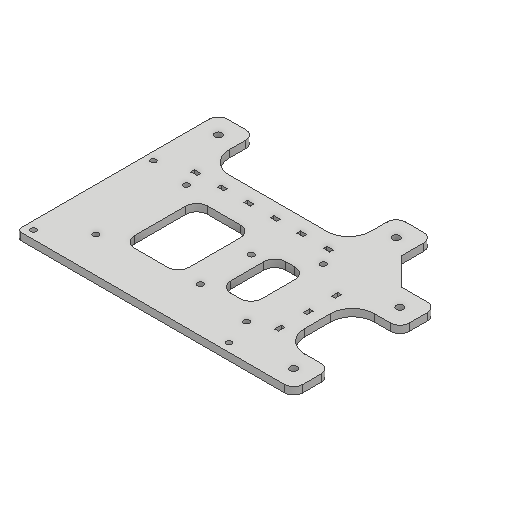
# Autodesk Inventor part: 3DP_PLA_Controller_Case_Bottom
Saved by Autodesk Inventor 2026.1 (Build 301233000, 233)
## iProperties
Created: 2017-05-26
Part Number: 3DP_PLA_Controller_Case_Bottom
Material: Ogólny
Document SubType Name: Modeling
Designer: Andrzej
Density: 1 g/cm^3
Appearance: Domyślna
Mass: 43.8091 g
Surface Area: 260.289 cm^2
Volume: 43.8091 cm^3
Author: Andrzej
Autodesk Inventor part; units mm, degrees
ref_plane "YZ Plane" through (0, 0, 0) normal (1, 0, 0) x (0, 1, 0)
ref_plane "XZ Plane" through (0, 0, 0) normal (0, 1, 0) x (-1, 0, 0)
ref_plane "XY Plane" through (0, 0, 0) normal (0, 0, 1) x (1, 0, 0)
sketch "Szkic1" plane through (0, 0, 0) normal (0, 0, 1) x (1, 0, 0)
  line L0 (0, 53.1646) -> (0, 0)
  line L1 (0, 0) -> (98.9175, 0)
  line L2 (98.9175, 0) -> (98.9175, 1.2597)
  line L3 (98.9175, 1.2597) -> (101.455, 3.8466)
  line L4 (101.455, 3.8466) -> (101.455, 38.0126)
  line L5 (101.455, 38.0126) -> (98.9175, 40.5017)
  line L6 (98.9175, 40.5017) -> (98.9175, 50.7051)
  line L7 (98.9175, 50.7051) -> (96.4101, 53.1646)
  line L8 (96.4101, 53.1646) -> (0, 53.1646)
  circle A0 centre (96.3111, 2.4061) radius 1.6
  circle A1 centre (15.0311, 50.6661) radius 1.6
  circle A2 centre (89.9611, 50.6661) radius 1.6
  circle A3 centre (13.7611, 2.4061) radius 1.6
  circle A4 centre (65.8311, 35.4261) radius 1.6
  circle A5 centre (65.8311, 7.4861) radius 1.6
  line L9 (-10, 93.1646) -> (141.455, 93.1646)
  line L10 (141.455, 93.1646) -> (141.455, -17)
  line L11 (141.455, -17) -> (-10, -17)
  line L12 (-10, -17) -> (-10, 93.1646)
  line L13 (107.455, 93.1646) -> (107.455, 61.1646)
  line L14 (107.455, 61.1646) -> (141.455, 61.1646)
  point P0 (-10, 13.9306)
  point P1 (7.9866, -17)
  dimension "d0" = 101.455
  dimension "d1" = 53.1646
  dimension "d2" = 98.9175
  dimension "d3" = 15.0311
  dimension "d4" = 2.4986
  dimension "d5" = 3.2
  dimension "d6" = 2.4986
  dimension "d7" = 8.9564
  dimension "d8" = 3.2
  dimension "d9" = 3.2
  dimension "d10" = 17.7386
  dimension "d11" = 65.8311
  dimension "d12" = 13.7611
  dimension "d13" = 2.4061
  dimension "d14" = 7.486
  dimension "d15" = 65.8311
  dimension "d16" = 2.4061
  dimension "d17" = 5.144
  dimension "d18" = 3.2
  dimension "d19" = 3.2
  dimension "d20" = 3.2
  dimension "d21" = 98.9175
  dimension "d22" = 1.2597
  dimension "d23" = 10.2034
  dimension "d24" = 34.166
  dimension "d33" = 40
  dimension "d34" = 40
  dimension "d35" = 17
  dimension "d36" = 10
  dimension "d37" = 34
  dimension "d38" = 32
  constraints: 30 end point, 6 centre point, 4 point on line, 2 parallel, 2 perpendicular, 1 horizontal, 1 vertical
  measures "d0" distance between parallel lines of L4 L0
  measures "d1" distance between parallel lines of L1 L8
  measures "d2" distance between parallel lines of L0 L6
  measures "d3" distance from line of L0 A1.centre
  measures "d4" distance from line of L8 A1.centre
  measures "d5" diameter of A1
  measures "d6" distance from line of L8 A2.centre
  measures "d7" distance from line of L6 A2.centre
  measures "d8" diameter of A2
  measures "d9" diameter of A4
  measures "d10" distance from line of L8 A4.centre
  measures "d11" distance from line of L0 A4.centre
  measures "d12" distance from line of L0 A3.centre
  measures "d13" distance from line of L1 A3.centre
  measures "d14" distance from line of L1 A5.centre
  measures "d15" distance from line of L0 A5.centre
  measures "d16" distance from line of L1 A0.centre
  measures "d17" distance from line of L4 A0.centre
  measures "d18" diameter of A0
  measures "d19" diameter of A5
  measures "d20" diameter of A3
  measures "d21" distance between parallel lines of L0 L2
  measures "d22" distance of L2.start L2.end
  measures "d23" distance of L5.end L6.end
  measures "d24" distance of L3.end L5.start
  measures "d33" distance between parallel lines of L10 L4
  measures "d34" distance between parallel lines of L9 L8
  measures "d35" distance between parallel lines of L1 L11
  measures "d36" distance between parallel lines of L12 L0
  measures "d37" distance between parallel lines of L10 L13
  measures "d38" distance between parallel lines of L14 L9
extrude "Wyciągnięcie proste1" add sketch "Szkic1" along normal blind 4 contours L8 L7 L6 L5 L4 L3 L2 L1 L0 | L9 L13 L14 L10 L11 L12
chamfer "Faza1" distance 15 angle 45 1 edges at (107.455, 61.1646, 2)
sketch "Szkic2" plane through (0, 0, 4) normal (0, 0, 1) x (1, 0, 0)
  circle A0 centre (65.8311, 7.4861) radius 1.6 projected
  circle A1 centre (15.0311, 50.6661) radius 1.6 projected
  circle A2 centre (89.9611, 50.6661) radius 1.6 projected
  circle A3 centre (13.7611, 2.4061) radius 1.6 projected
  circle A4 centre (65.8311, 35.4261) radius 1.6 projected
  circle A5 centre (96.3111, 2.4061) radius 1.6 projected
  line L0 (-10, 93.1646) -> (-10, -17) projected
  line L1 (-10, -17) -> (141.455, -17) projected
  line L2 (141.455, -17) -> (141.455, 61.1646) projected
  line L3 (141.455, 61.1646) -> (122.455, 61.1646) projected
  line L4 (107.455, 76.1646) -> (122.455, 61.1646) projected
  line L5 (107.455, 76.1646) -> (107.455, 93.1646) projected
  line L6 (107.455, 93.1646) -> (-10, 93.1646) projected
  line L7 (10, 93.1646) -> (10, 67.1646)
  line L8 (10, 67.1646) -> (87.455, 67.1646)
  line L9 (87.455, 67.1646) -> (87.455, 93.1646)
  line L10 (107.455, 93.1646) -> (-10, 93.1646) projected
  line L11 (141.455, -17) -> (141.455, 61.1646) projected
  line L12 (141.455, 41.1646) -> (115.455, 41.1646)
  line L13 (115.455, 41.1646) -> (115.455, 3)
  line L14 (115.455, 3) -> (141.455, 3)
  line L15 (10, 60.1646) -> (13.5, 60.1646)
  line L16 (13.5, 60.1646) -> (13.5, 58.1646)
  line L17 (13.5, 58.1646) -> (10, 58.1646)
  line L18 (10, 58.1646) -> (10, 60.1646)
  line L19 (28, 58.1646) -> (24.5, 58.1646)
  line L20 (28, 60.1646) -> (28, 58.1646)
  line L21 (24.5, 60.1646) -> (28, 60.1646)
  line L22 (24.5, 58.1646) -> (24.5, 60.1646)
  line L23 (42.5, 58.1646) -> (39, 58.1646)
  line L24 (42.5, 60.1646) -> (42.5, 58.1646)
  line L25 (39, 60.1646) -> (42.5, 60.1646)
  line L26 (39, 58.1646) -> (39, 60.1646)
  line L27 (57, 58.1646) -> (53.5, 58.1646)
  line L28 (57, 60.1646) -> (57, 58.1646)
  line L29 (53.5, 60.1646) -> (57, 60.1646)
  line L30 (53.5, 58.1646) -> (53.5, 60.1646)
  line L31 (71.5, 58.1646) -> (68, 58.1646)
  line L32 (71.5, 60.1646) -> (71.5, 58.1646)
  line L33 (68, 60.1646) -> (71.5, 60.1646)
  line L34 (68, 58.1646) -> (68, 60.1646)
  line L35 (86, 58.1646) -> (82.5, 58.1646)
  line L36 (86, 60.1646) -> (86, 58.1646)
  line L37 (82.5, 60.1646) -> (86, 60.1646)
  line L38 (82.5, 58.1646) -> (82.5, 60.1646)
  line L39 (109.455, 41.1646) -> (107.455, 41.1646)
  line L40 (107.455, 41.1646) -> (107.455, 37.6646)
  line L41 (107.455, 37.6646) -> (109.455, 37.6646)
  line L42 (109.455, 37.6646) -> (109.455, 41.1646)
  line L43 (107.455, 25.6646) -> (107.455, 22.1646)
  line L44 (107.455, 22.1646) -> (109.455, 22.1646)
  line L45 (109.455, 22.1646) -> (109.455, 25.6646)
  line L46 (109.455, 25.6646) -> (107.455, 25.6646)
  line L47 (107.455, 10.1646) -> (107.455, 6.6646)
  line L48 (107.455, 6.6646) -> (109.455, 6.6646)
  line L49 (109.455, 6.6646) -> (109.455, 10.1646)
  line L50 (109.455, 10.1646) -> (107.455, 10.1646)
  line L51 (54.7961, 6.5361) -> (24.7961, 6.5361)
  line L52 (24.7961, 6.5361) -> (24.7961, 46.5361)
  line L53 (24.7961, 46.5361) -> (54.7961, 46.5361)
  line L54 (54.7961, 46.5361) -> (54.7961, 6.5361)
  line L55 (89.5711, 11.5361) -> (72.5711, 11.5361)
  line L56 (72.5711, 11.5361) -> (72.5711, 41.5361)
  line L57 (72.5711, 41.5361) -> (89.5711, 41.5361)
  line L58 (89.5711, 41.5361) -> (89.5711, 11.5361)
  point P0 (0, 0)
  point P1 (131.455, -7)
  point P2 (131.455, 51.1646)
  point P3 (97.455, 83.1646)
  point P4 (0, 83.1646)
  dimension "d42" = 20
  dimension "d43" = 20
  dimension "d44" = 20
  dimension "d45" = 20
  dimension "d46" = 26
  dimension "d47" = 26
  dimension "d50" = 3.5
  dimension "d51" = 2
  dimension "d52" = 7
  dimension "d55" = 14.5
  dimension "d62" = 2
  dimension "d63" = 3.5
  dimension "d64" = 6
  dimension "d67" = 15.5
  dimension "d74" = 40
  dimension "d75" = 30
  dimension "d78" = 10
  dimension "d79" = 10
  dimension "d80" = 10
  dimension "d81" = 10
  dimension "d82" = 10
  dimension "d83" = 10
  dimension "d84" = 10
  dimension "d85" = 10
  dimension "d93" = 52.07
  dimension "d94" = 11.035
  dimension "d95" = 48.26
  dimension "d96" = 4.13
  dimension "d98" = 30
  dimension "d99" = 17
  dimension "d100" = 48.26
  dimension "d101" = 30.48
  dimension "d102" = 9.13
  dimension "d103" = 6.74
  constraints: 100 end point, 8 parallel, 8 perpendicular, 6 horizontal, 4 point on line, 2 collinear, 2 vertical, 56 other
  measures "d42" distance between parallel lines of L0 L7
  measures "d43" distance between parallel lines of L5 L9
  measures "d44" distance between parallel lines of L3 L12
  measures "d45" distance between parallel lines of L1 L14
  measures "d46" distance between parallel lines of L6 L8
  measures "d47" distance between parallel lines of L2 L13
  measures "d50" distance of L16.end L17.end
  measures "d51" distance of L15.end L16.end
  measures "d52" distance between parallel lines of L8 L15
  measures "d55" distance of L16.end L19.start
  measures "d62" distance of L41.end L40.end
  measures "d63" distance of L40.end L39.end
  measures "d64" distance between parallel lines of L13 L42
  measures "d67" distance of L39.end L43.start
  measures "d74" distance between parallel lines of L53 L51
  measures "d75" distance between parallel lines of L52 L54
  measures "d78" distance from line of L14 point (131.455, -7)
  measures "d79" distance from line of L3 point (131.455, 51.165)
  measures "d80" distance from line of L9 point (97.455, 83.165)
  measures "d81" distance from line of L7 point (0, 83.165)
  measures "d82" distance from line of L2 point (131.455, -7)
  measures "d83" distance from line of L2 point (131.455, 51.165)
  measures "d84" distance from line of L6 point (97.455, 83.165)
  measures "d85" distance from line of L10 point (0, 83.165)
  measures "d93" horizontal distance of A3.centre A0.centre
  measures "d94" distance from line of L54 A0.centre
  measures "d95" vertical distance of A1.centre A3.centre
  measures "d96" distance from line of A1.centre L53
  measures "d98" distance between parallel lines of L55 L57
  measures "d99" distance between parallel lines of L56 L58
  measures "d100" vertical distance of A2.centre A5.centre
  measures "d101" horizontal distance of A0.centre A5.centre
  measures "d102" distance from line of A5.centre L55
  measures "d103" distance from line of A0.centre L56
extrude "Wyciągnięcie proste3" cut sketch "Szkic2" against normal through all contours L6 L9 L8 L7 | L14 L13 L12 L2 | L15 L16 L17 L18 | L19 L22 L21 L20 | L23 L26 L25 L24 | L27 L30 L29 L28 | L31 L34 L33 L32 | L35 L38 L37 L36 | L42 L41 L40 L39 | L46 L45 L44 L43 | L50 L49 L48 L47 | L51 L52 L53 L54 | L55 L56 L57 L58
fillet "Zaokrąglenie1" radius 12 4 edges at (115.455, 41.1646, 2) (115.455, 3, 2) (87.455, 67.1646, 2) (10, 67.1646, 2)
fillet "Zaokrąglenie1" radius 5 8 edges at (10, 93.1646, 2) (-10, 93.1646, 2) (87.455, 93.1646, 2) (107.455, 93.1646, 2) (141.455, 61.1646, 2) (141.455, 41.1646, 2) (141.455, 3, 2) (141.455, -17, 2)
hole "Otwór1" at (131.455, -7, 4) at (131.455, 51.1646, 4) at (97.455, 83.1646, 4) at (0, 83.1646, 4) direction (0, 0, -1) diameter 4 end through all
fillet "Zaokrąglenie2" radius 6 8 edges at (24.7961, 6.5361, 2) (24.7961, 46.5361, 2) (54.7961, 46.5361, 2) (54.7961, 6.5361, 2) (89.5711, 11.5361, 2) (89.5711, 41.5361, 2) (72.5711, 41.5361, 2) (72.5711, 11.5361, 2)
fillet "Zaokrąglenie2" radius 2 1 edges at (-10, -17, 2)
sketch "Szkic4" plane through (0, 0, 4) normal (0, 0, 1) x (1, 0, 0)
  arc A0 (-10, -15) -> (-8, -17) centre (-8, -15) ccw projected
  line L0 (-8, -17) -> (136.455, -17) projected
  arc A1 (136.455, -17) -> (141.455, -12) centre (136.455, -12) ccw projected
  line L1 (141.455, -12) -> (141.455, -2) projected
  arc A2 (141.455, -2) -> (136.455, 3) centre (136.455, -2) ccw projected
  line L2 (136.455, 3) -> (127.455, 3) projected
  arc A3 (115.455, 15) -> (127.455, 3) centre (127.455, 15) ccw projected
  line L3 (115.455, 15) -> (115.455, 29.1646) projected
  arc A4 (127.455, 41.1646) -> (115.455, 29.1646) centre (127.455, 29.1646) ccw projected
  line L4 (127.455, 41.1646) -> (136.455, 41.1646) projected
  arc A5 (136.455, 41.1646) -> (141.455, 46.1646) centre (136.455, 46.1646) ccw projected
  line L5 (141.455, 46.1646) -> (141.455, 56.1646) projected
  arc A6 (141.455, 56.1646) -> (136.455, 61.1646) centre (136.455, 56.1646) ccw projected
  line L6 (136.455, 61.1646) -> (122.455, 61.1646) projected
  line L7 (107.455, 76.1646) -> (122.455, 61.1646) projected
  line L8 (107.455, 76.1646) -> (107.455, 88.1646) projected
  arc A7 (107.455, 88.1646) -> (102.455, 93.1646) centre (102.455, 88.1646) ccw projected
  line L9 (102.455, 93.1646) -> (92.455, 93.1646) projected
  arc A8 (92.455, 93.1646) -> (87.455, 88.1646) centre (92.455, 88.1646) ccw projected
  line L10 (87.455, 88.1646) -> (87.455, 79.1646) projected
  arc A9 (75.455, 67.1646) -> (87.455, 79.1646) centre (75.455, 79.1646) ccw projected
  line L11 (75.455, 67.1646) -> (22, 67.1646) projected
  arc A10 (10, 79.1646) -> (22, 67.1646) centre (22, 79.1646) ccw projected
  line L12 (10, 79.1646) -> (10, 88.1646) projected
  arc A11 (10, 88.1646) -> (5, 93.1646) centre (5, 88.1646) ccw projected
  line L13 (5, 93.1646) -> (-5, 93.1646) projected
  arc A12 (-5, 93.1646) -> (-10, 88.1646) centre (-5, 88.1646) ccw projected
  line L14 (-10, 88.1646) -> (-10, -15) projected
  circle A13 centre (97.455, 83.1646) radius 2 projected
  circle A14 centre (131.455, -7) radius 2 projected
  circle A15 centre (131.455, 51.1646) radius 2 projected
  circle A16 centre (0, 83.1646) radius 2 projected
  line L15 (89.5711, 35.5361) -> (89.5711, 17.5361) projected
  arc A17 (83.5711, 11.5361) -> (89.5711, 17.5361) centre (83.5711, 17.5361) ccw projected
  line L16 (83.5711, 11.5361) -> (78.5711, 11.5361) projected
  arc A18 (72.5711, 17.5361) -> (78.5711, 11.5361) centre (78.5711, 17.5361) ccw projected
  line L17 (72.5711, 17.5361) -> (72.5711, 35.5361) projected
  arc A19 (78.5711, 41.5361) -> (72.5711, 35.5361) centre (78.5711, 35.5361) ccw projected
  line L18 (78.5711, 41.5361) -> (83.5711, 41.5361) projected
  arc A20 (89.5711, 35.5361) -> (83.5711, 41.5361) centre (83.5711, 35.5361) ccw projected
  line L19 (107.455, 22.1646) -> (107.455, 25.6646) projected
  line L20 (107.455, 25.6646) -> (109.455, 25.6646) projected
  line L21 (109.455, 25.6646) -> (109.455, 22.1646) projected
  line L22 (109.455, 22.1646) -> (107.455, 22.1646) projected
  line L23 (82.5, 60.1646) -> (86, 60.1646) projected
  line L24 (86, 60.1646) -> (86, 58.1646) projected
  line L25 (86, 58.1646) -> (82.5, 58.1646) projected
  line L26 (82.5, 58.1646) -> (82.5, 60.1646) projected
  line L27 (53.5, 60.1646) -> (57, 60.1646) projected
  line L28 (57, 60.1646) -> (57, 58.1646) projected
  line L29 (57, 58.1646) -> (53.5, 58.1646) projected
  line L30 (53.5, 58.1646) -> (53.5, 60.1646) projected
  line L31 (24.5, 60.1646) -> (28, 60.1646) projected
  line L32 (28, 60.1646) -> (28, 58.1646) projected
  line L33 (28, 58.1646) -> (24.5, 58.1646) projected
  line L34 (24.5, 58.1646) -> (24.5, 60.1646) projected
  line L35 (10, 58.1646) -> (10, 60.1646) projected
  line L36 (10, 60.1646) -> (13.5, 60.1646) projected
  line L37 (13.5, 60.1646) -> (13.5, 58.1646) projected
  line L38 (13.5, 58.1646) -> (10, 58.1646) projected
  line L39 (39, 60.1646) -> (42.5, 60.1646) projected
  line L40 (42.5, 60.1646) -> (42.5, 58.1646) projected
  line L41 (42.5, 58.1646) -> (39, 58.1646) projected
  line L42 (39, 58.1646) -> (39, 60.1646) projected
  line L43 (68, 60.1646) -> (71.5, 60.1646) projected
  line L44 (71.5, 60.1646) -> (71.5, 58.1646) projected
  line L45 (71.5, 58.1646) -> (68, 58.1646) projected
  line L46 (68, 58.1646) -> (68, 60.1646) projected
  line L47 (107.455, 37.6646) -> (107.455, 41.1646) projected
  line L48 (107.455, 41.1646) -> (109.455, 41.1646) projected
  line L49 (109.455, 41.1646) -> (109.455, 37.6646) projected
  line L50 (109.455, 37.6646) -> (107.455, 37.6646) projected
  line L51 (107.455, 6.6646) -> (107.455, 10.1646) projected
  line L52 (107.455, 10.1646) -> (109.455, 10.1646) projected
  line L53 (109.455, 10.1646) -> (109.455, 6.6646) projected
  line L54 (109.455, 6.6646) -> (107.455, 6.6646) projected
  line L55 (54.7961, 40.5361) -> (54.7961, 12.5361) projected
  arc A21 (48.7961, 6.5361) -> (54.7961, 12.5361) centre (48.7961, 12.5361) ccw projected
  line L56 (48.7961, 6.5361) -> (30.7961, 6.5361) projected
  arc A22 (24.7961, 12.5361) -> (30.7961, 6.5361) centre (30.7961, 12.5361) ccw projected
  line L57 (24.7961, 12.5361) -> (24.7961, 40.5361) projected
  arc A23 (30.7961, 46.5361) -> (24.7961, 40.5361) centre (30.7961, 40.5361) ccw projected
  line L58 (30.7961, 46.5361) -> (48.7961, 46.5361) projected
  arc A24 (54.7961, 40.5361) -> (48.7961, 46.5361) centre (48.7961, 40.5361) ccw projected
  circle A25 centre (65.8311, 7.4861) radius 1.6 projected
  circle A26 centre (15.0311, 50.6661) radius 1.6 projected
  circle A27 centre (89.9611, 50.6661) radius 1.6 projected
  circle A28 centre (13.7611, 2.4061) radius 1.6 projected
  circle A29 centre (65.8311, 35.4261) radius 1.6 projected
  circle A30 centre (96.3111, 2.4061) radius 1.6 projected
  point P0 (0, 0)
  point P1 (-5.5, 53.1646)
  point P2 (-5.5, -12.5)
  point P3 (101.455, -12.5)
  dimension "d105" = 40
  dimension "d106" = 40
  dimension "d107" = 4.5
  dimension "d108" = 4.5
  dimension "d109" = 4.5
  dimension "d110" = 4.5
  measures "d105" distance from line of point (-5.5, 53.165) L13
  measures "d106" distance from line of L1 point (101.455, -12.5)
  measures "d107" distance from line of L14 point (-5.5, 53.165)
  measures "d108" distance from line of L0 point (101.455, -12.5)
  measures "d109" distance from line of L0 point (-5.5, -12.5)
  measures "d110" distance from line of L14 point (-5.5, -12.5)
hole "Otwór2" at (-5.5, 53.1646, 4) at (-5.5, -12.5, 4) at (101.455, -12.5, 4) direction (0, 0, -1) diameter 3 end through all
equation "\"d47\" = d46"
equation "\"d94\" = -0.5 * d75 + 0.5 * d93"
equation "\"d96\" = -0.5 * d74 + 0.5 * d95"
equation "\"d102\" = -0.5 * d98 + 0.5 * d100"
equation "\"d103\" = -0.5 * d99 + 0.5 * d101"
equation "\"d106\" = d105"
equation "\"d107\" = d110"
equation "\"d108\" = d110"
equation "\"d109\" = d110"
